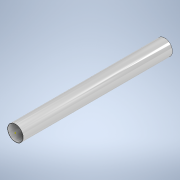
# Autodesk Inventor part: Barra
Saved by Autodesk Inventor 2020 (Build 240168000, 168)
## iProperties
Created: 2019-09-24
Part Number: Barra
Material: Aluminio 6061-AHC
Document SubType Name: Modeling
Designer: Frederich Schnëider
Density: 2.7 g/cm^3
Appearance: Aluminio - Oscuro
Author: Frederich Schnëider
Autodesk Inventor part; units mm, degrees
ref_plane "YZ Plane" through (0, 0, 0) normal (1, 0, 0) x (0, 1, 0)
ref_plane "XZ Plane" through (0, 0, 0) normal (0, 1, 0) x (-1, 0, 0)
ref_plane "XY Plane" through (0, 0, 0) normal (0, 0, 1) x (1, 0, 0)
sketch "Boceto1" plane through (0, 0, 0) normal (0, 0, 1) x (1, 0, 0)
  circle A0 centre (0, 0) radius 2.9
  dimension "d0" = 5.8
  constraints: 1 centre point, 1 coincident
  measures "d0" diameter of A0
extrude "Extrusión1" add sketch "Boceto1" along normal blind 55
sketch "Boceto2" plane through (0, 0, 55) normal (0, 0, 1) x (1, 0, 0)
  point P0 (0, 0)
sketch "Boceto3" plane through (0, 0, 55) normal (0, 0, 1) x (1, 0, 0)
  circle A0 centre (0, 0) radius 2.8
  dimension "d3" = 5.6
  constraints: 1 centre point, 1 coincident
  measures "d3" diameter of A0
extrude "Extrusión2" cut sketch "Boceto3" against normal blind 57.9
